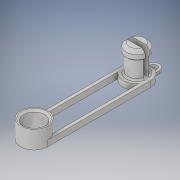
# Autodesk Inventor part: link_v2ipt
Saved by Autodesk Inventor 2019 (Build 230136000, 136)
## iProperties
Created: 2020-06-08
Part Number: link_v2ipt
Material: Genérico
Document SubType Name: Modeling
Designer: Samuel
Density: 1 g/cm^3
Appearance: Valor por defecto
Author: Samuel
Autodesk Inventor part; units mm, degrees
note: some values were not read from the file. Chosen so that the rebuilt part matches the saved one: sketch regions of "Extrusión1".
ref_plane "YZ Plane" through (0, 0, 0) normal (1, 0, 0) x (0, 1, 0)
ref_plane "XZ Plane" through (0, 0, 0) normal (0, 1, 0) x (-1, 0, 0)
ref_plane "XY Plane" through (0, 0, 0) normal (0, 0, 1) x (1, 0, 0)
sketch "Boceto1" plane through (0, 0, 0) normal (0, 1, 0) x (-1, 0, 0)
  line L0 (45, 172) -> (-45, 172)
  line L1 (-45, 172) -> (-45, -172)
  line L2 (-45, -172) -> (45, -172)
  line L3 (45, -172) -> (45, 172)
  line L4 (45, 172) -> (-45, -172) construction
  line L5 (-45, 172) -> (45, -172) construction
  circle A0 centre (0, -172) radius 45
  circle A1 centre (0, 172) radius 45
  circle A2 centre (0, 172) radius 34.798
  line L6 (45, 172) -> (-45, 172)
  point P0 (0, 0)
  dimension "d0" = 90
  dimension "d1" = 344
  dimension "d2" = 90
  dimension "d3" = 90
  dimension "d4" = 69.596
  constraints: 14 end point, 4 midpoint, 3 centre point, 3 equal length, 1 coincident, 1 horizontal, 1 perpendicular
  measures "d0" distance of L2.end L1.end
  measures "d1" distance of L1.end L0.end
  measures "d2" diameter of A0
  measures "d3" diameter of A1
  measures "d4" diameter of A2
extrude "Extrusión1" add sketch "Boceto1" along normal blind 20 contours A1 L0 A2 | L0 A2 A1 | L3 A0 L1 A1 | A2 L0 | A0 L2 | L2 A0 picked at (9.4719, 153.1181)
sketch "Boceto3" plane through (0, 20, 0) normal (0, 1, 0) x (1, 0, 0)
  line L0 (34.798, -172) -> (-34.798, -172) projected
  circle A0 centre (0, -172) radius 34.798
  point P0 (0, 0)
  constraints: 1 centre point, 1 midpoint
extrude "Extrusión2" cut sketch "Boceto3" against normal blind 20
sketch "Boceto5" plane through (0, 20, 0) normal (0, 1, 0) x (1, 0, 0)
  circle A0 centre (0, -172) radius 34.798 projected
  line L0 (-45, 172) -> (-45, -172) projected
  arc A1 (-45, -172) -> (45, -172) centre (0, -172) ccw projected
  line L1 (45, -172) -> (45, 172) projected
  arc A2 (45, 172) -> (-45, 172) centre (0, 172) ccw projected
  line L2 (34.798, -172) -> (-34.798, 172) construction
  line L3 (-34.798, -172) -> (34.798, 172) construction
  line L4 (-45, 172) -> (-45, -172) projected
  arc A3 (34.798, -143.4676) -> (-34.798, -143.4676) centre (0, -172) ccw
  arc A4 (-34.798, 143.4676) -> (34.798, 143.4676) centre (0, 172) ccw
  line L5 (-34.798, -143.4676) -> (-34.798, 143.4676)
  line L6 (34.798, 143.4676) -> (34.798, -143.4676)
  line L7 (45, -172) -> (45, 172) projected
  point P0 (0, 0)
  constraints: 8 end point, 4 point on circle, 2 centre point, 2 coincident, 2 midpoint, 2 parallel
extrude "Extrusión3" cut sketch "Boceto5" against normal blind 20 contours A3 L5 A4 L6
sketch "Boceto6" plane through (0, 20, 0) normal (0, 1, 0) x (1, 0, 0)
  circle A0 centre (0, -172) radius 34.798 projected
  arc A1 (34.798, -143.4676) -> (-34.798, -143.4676) centre (0, -172) ccw projected
  arc A2 (-45, -172) -> (45, -172) centre (0, -172) ccw projected
  arc A3 (-34.798, 143.4676) -> (34.798, 143.4676) centre (0, 172) ccw projected
  circle A4 centre (0, -172) radius 34.798
  circle A5 centre (0, -172) radius 45
  circle A6 centre (0, 172) radius 45
  point P0 (0, 0)
  constraints: 4 coincident, 3 centre point, 2 concentric
extrude "Extrusión4" add sketch "Boceto6" along normal blind 40.35 contours A5 A2 A1
chamfer "Chaflán1" distance 6.35 angle 45 2 edges at (-34.798, 60.35, 172) (34.798, 0, 172)
sketch "Boceto7" plane through (0, 20, 0) normal (0, 1, 0) x (1, 0, 0)
  arc A0 (-34.798, -143.4676) -> (-45, -172) centre (0, -172) ccw projected
  line L0 (-34.798, -143.4676) -> (-34.798, 143.4676) projected
  arc A1 (-34.798, 143.4676) -> (34.798, 143.4676) centre (0, 172) ccw projected
  line L1 (34.798, 143.4676) -> (34.798, -143.4676) projected
  arc A2 (45, -172) -> (34.798, -143.4676) centre (0, -172) ccw projected
  line L2 (45, -172) -> (45, 172) projected
  arc A3 (45, 172) -> (-45, 172) centre (0, 172) ccw projected
  line L3 (-45, 172) -> (-45, -172) projected
  circle A4 centre (0, 172) radius 30.48
  point P0 (0, 0)
  dimension "d16" = 60.96
  constraints: 1 centre point, 1 coincident
  measures "d16" diameter of A4
extrude "Extrusión5" add sketch "Boceto7" along normal blind 88.9 contours A4
sketch "Boceto9" plane through (0, 108.9, -172) normal (0, 1, 0) x (1, 0, 0)
  circle A0 centre (0, 0) radius 36
  point P0 (0, -172)
  dimension "d20" = 72
  constraints: 1 centre point
  measures "d20" diameter of A0
extrude "Extrusión6" add sketch "Boceto9" against normal blind 30.48
chamfer "Chaflán2" distance 10.56 angle 45 1 edges at (-36, 108.9, -172)
chamfer "Chaflán3" distance 5.08 angle 45 1 edges at (-36, 78.42, -172)
fillet "Empalme1" radius 5 1 edges at (-30.48, 20, -172)
sketch "Boceto10" plane through (0, 108.9, -172) normal (0, 1, 0) x (1, 0, 0)
  circle A0 centre (0, 0) radius 25.44 projected
  arc A1 (45, 0) -> (-45, 0) centre (0, 0) ccw projected
  line L0 (44.3276, -7.75) -> (-44.3276, -7.75)
  line L1 (-44.3276, -7.75) -> (-44.3276, 7.75)
  line L2 (-44.3276, 7.75) -> (44.3276, 7.75)
  line L3 (44.3276, 7.75) -> (44.3276, -7.75)
  line L4 (44.3276, -7.75) -> (-44.3276, 7.75) construction
  line L5 (-44.3276, -7.75) -> (44.3276, 7.75) construction
  point P0 (0, -172)
  dimension "d30" = 15.5
  constraints: 12 end point, 2 midpoint, 2 parallel, 1 horizontal, 1 perpendicular, 1 point on circle
  measures "d30" distance of L0.end L1.end
extrude "Extrusión7" cut sketch "Boceto10" against normal blind 88.9 contours A0 L0 L2 | A0 L2 L3 L0 | A0 L0 L1 L2
ref_plane "Plano de trabajo1" through (0, 0, -217) normal (0, 0, -1) x (-1, 0, 0)
sketch "Boceto11" plane through (0, 0, -217) normal (0, 0, -1) x (-1, 0, 0)
  line L0 (45, 0) -> (45, 20) projected
  line L1 (-45, 20) -> (45, 20) projected
  line L2 (-45, 20) -> (-45, 0) projected
  line L3 (-45, 0) -> (45, 0) projected
  line L4 (45, 0) -> (-45, 0) projected
  line L5 (-20, 20) -> (20, 20)
  line L6 (20, 20) -> (20, 0)
  line L7 (20, 0) -> (-20, 0)
  line L8 (-20, 0) -> (-20, 20)
  line L9 (-20, 20) -> (20, 0) construction
  line L10 (20, 20) -> (-20, 0) construction
  point P0 (0, 0)
  point P1 (0, 10)
  constraints: 12 end point, 2 midpoint, 2 parallel, 1 horizontal, 1 perpendicular, 1 point on line
extrude "Extrusión8" add sketch "Boceto11" along normal blind 30 and the other way blind 10 contours L3 L8 L1 L6
sketch "Boceto15" plane through (0, 20, 0) normal (0, 1, 0) x (1, 0, 0)
  arc A0 (-20, 212.3113) -> (-45, 172) centre (0, 172) ccw projected
  line L0 (-45, 172) -> (-45, -172) projected
  arc A1 (-34.798, -143.4676) -> (-45, -172) centre (0, -172) ccw projected
  line L1 (-34.798, -143.4676) -> (-34.798, 143.4676) projected
  arc A2 (-34.798, 143.4676) -> (34.798, 143.4676) centre (0, 172) ccw projected
  line L2 (34.798, 143.4676) -> (34.798, -143.4676) projected
  arc A3 (45, -172) -> (34.798, -143.4676) centre (0, -172) ccw projected
  line L3 (45, -172) -> (45, 172) projected
  arc A4 (45, 172) -> (20, 212.3113) centre (0, 172) ccw projected
  line L4 (20, 212.3113) -> (20, 247) projected
  line L5 (-20, 247) -> (20, 247) projected
  line L6 (-20, 212.3113) -> (-20, 247) projected
  arc A5 (34.6232, 179.75) -> (-34.6232, 179.75) centre (0, 172) ccw projected
  line L7 (-34.6232, 179.75) -> (34.6232, 179.75) projected
  line L8 (34.6232, 164.25) -> (-34.6232, 164.25) projected
  arc A6 (-34.6232, 164.25) -> (34.6232, 164.25) centre (0, 172) ccw projected
  arc A7 (12, 227) -> (-12, 227) centre (0, 227) ccw
  line L9 (12, 227) -> (12, 212.3113)
  line L10 (-12, 227) -> (-12, 212.3113)
  arc A8 (45, 172) -> (20, 212.3113) centre (0, 172) ccw projected
  line L11 (-20, 227) -> (-20, 247)
  line L12 (20, 247) -> (-20, 247) projected
  line L13 (-20, 247) -> (20, 247)
  line L14 (20, 247) -> (20, 227)
  line L15 (-12, 212.3113) -> (12, 212.3113)
  line L16 (-20, 227) -> (-20, 247)
  line L17 (20, 247) -> (0, 247)
  line L18 (-20, 247) -> (0, 247)
  line L19 (-20, 247) -> (-20, 227)
  arc A9 (20, 227) -> (0, 247) centre (0, 227) ccw
  arc A10 (0, 247) -> (-20, 227) centre (0, 227) ccw
  line L20 (20, 212.3113) -> (20, 247) projected
  line L21 (20, 227) -> (20, 247)
  line L22 (20, 247) -> (0, 247)
  point P0 (0, 0)
  constraints: 24 end point, 6 point on circle, 3 centre point, 2 coincident, 2 collinear, 2 horizontal, 2 perpendicular, 1 parallel, 1 point on line, 1 tangent, 1 vertical
extrude "Extrusión11" cut sketch "Boceto15" against normal blind 50 contours L6 L5 A10 | L5 L4 A9 | L9 L15 L10 A7
sketch "Boceto16" plane through (20, 0, -212.3113) normal (1, 0, 0) x (0, 0, -1)
  line L0 (14.6887, 0) -> (14.6887, 20) projected
  line L1 (0, 20) -> (14.6887, 20) projected
  line L2 (0, 0) -> (0, 20) projected
  line L3 (0, 0) -> (14.6887, 0) projected
  line L4 (0, 20) -> (38, 20)
  line L5 (38, 20) -> (38, 9)
  line L6 (38, 9) -> (0, 9)
  line L7 (0, 9) -> (0, 20)
  point P0 (-212.3113, 0)
  constraints: 8 end point, 2 parallel, 1 horizontal, 1 perpendicular
extrude "Extrusión12" cut sketch "Boceto16" against normal blind 50 contours L6 L2 L1 L0 | L0 L4 L5 L6
